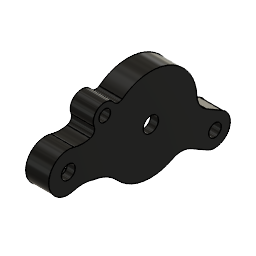
Dribbler Gear Cover v1 (Autodesk Fusion 360 design; units mm, degrees)
part number: 2026-04-20-20-56-39-992
Autodesk Fusion 360 part; units mm, degrees
sketch "Sketch1" plane through (0, 0, 0) normal (1, 0, 0) x (0, 0, -1)
  circle A0 centre (0, 0) radius 12
  circle A1 centre (0, 0) radius 2
  line L0 (0, 0) -> (-13.9, 0)
  circle A2 centre (-13.9, 0) radius 5.1
  line L1 (0, 0) -> (-21.5, 0)
  circle A3 centre (-21.5, 0) radius 5.1
  circle A4 centre (-21.5, 0) radius 1.8
  circle A5 centre (-13.9, 0) radius 1.75
  dimension "d1" = 24
  dimension "d3" = 4
  dimension "d4" = 13.9
  dimension "d5" = 10.2
  dimension "d6" = 21.5
  dimension "d7" = 10.2
  dimension "d8" = 3.6
  dimension "d9" = 3.5
  constraint coincident A0.centre A1.centre
  constraint horizontal L0
  constraint coincident L0.end A2.centre
  constraint parallel L0 L1
  constraint coincident L1.end A3.centre
  constraint concentric A3 A4
  constraint concentric A2 A5
  measures "d1" diameter of A0
  measures "d3" diameter of A1
  measures "d4" distance of A0.centre L0.end
  measures "d5" diameter of A2
  measures "d6" distance of A0.centre L1.end
  measures "d7" diameter of A3
  measures "d8" diameter of A4
  measures "d9" diameter of A5
extrude "Extrude1" add sketch "Sketch1" against normal blind 2 contours A0 A2 | A0 L0 A2 L1 | A0 L0 A2 L1 A3 A5 | A0 L0 A2 L1 A3 A5 | A0 L0 A2 L1 | A2 L1 A3 | A2 A3 | A2 L1 A3
extrude "Extrude2" add sketch "Sketch1" against normal blind 6 contours L0 L1 A5 | L0 L1 A5
fillet "Fillet1" radius 10 2 edges at (-1, 4.3231, 11.1942) (-1, -4.3231, 11.1942)
fillet "Fillet2" radius 8 2 edges at (-1, -3.4015, 17.7) (-1, 3.4015, 17.7)
sketch "Sketch2" plane through (-2, 0, 0) normal (-1, 0, 0) x (0, 0, 1)
  circle A0 centre (21.5, 0) radius 1.8
  circle A1 centre (13.9, 0) radius 1.75
  circle A2 centre (0, 0) radius 2
  arc A3 (15.3794, 4.8807) -> (14.6627, 5.0426) centre (13.9, 0) ccw
  arc A4 (8.8136, 8.1437) -> (14.6627, 5.0426) centre (16.1583, 14.9302) ccw
  arc A5 (8.8136, 8.1437) -> (8.8136, -8.1437) centre (0, 0) ccw
  arc A6 (14.6627, -5.0426) -> (8.8136, -8.1437) centre (16.1583, -14.9302) ccw
  arc A7 (14.6627, -5.0426) -> (15.3794, -4.8807) centre (13.9, 0) ccw
  arc A8 (20.0206, -4.8807) -> (15.3794, -4.8807) centre (17.7, -12.5367) ccw
  arc A9 (20.0206, -4.8807) -> (20.0206, 4.8807) centre (21.5, 0) ccw
  arc A10 (15.3794, 4.8807) -> (20.0206, 4.8807) centre (17.7, 12.5367) ccw
  circle A11 centre (0, 0) radius 11
  circle A12 centre (0, 0) radius 12
  circle A13 centre (13.9, 0) radius 4.6
  circle A14 centre (21.5, 0) radius 4.6
  circle A15 centre (13.9, 0) radius 5.1
  circle A16 centre (21.5, 0) radius 5.1
  dimension "d18" = 22
  dimension "d19" = 9.2
  dimension "d20" = 9.2
  dimension "d21" = 10.2
  dimension "d22" = 10.2
  constraint concentric A2 A11
  constraint concentric A11 A12
  constraint concentric A1 A13
  constraint concentric A0 A14
  constraint concentric A13 A15
  constraint concentric A14 A16
  measures "d18" diameter of A11
  measures "d19" diameter of A13
  measures "d20" diameter of A14
  measures "d21" diameter of A15
  measures "d22" diameter of A16
extrude "Extrude3" add sketch "Sketch2" along normal blind 4 contours A3 A12 A13 A15 A16 | A10 A15 A16 | A4 A12 A15 | A9 A14 A15 A16 | A5 A11 A12 A15 | A6 A12 A15 | A8 A15 A16 | A7 A12 A13 A15 A16
fillet "Fillet3" radius 4 1 edges at (-4, 3.6779, 10.3669)
fillet "Fillet4" radius 6 1 edges at (-4, 3.8409, 11.3687)
fillet "Fillet5" radius 4 1 edges at (-4, -3.6779, 10.3669)
fillet "Fillet6" radius 6 1 edges at (-4, -3.8409, 11.3687)
fillet "Fillet7" radius 15 4 edges at (-4, -3.0072, 17.3809) (-4, -3.0072, 18.0191) (-4, 3.0072, 17.3809) (-4, 3.0072, 18.0191)
sketch "Sketch3" plane through (0, 0, 0) normal (1, 0, 0) x (0, 0, -1)
  circle A0 centre (0, 0) radius 2
  circle A1 centre (-21.5, 0) radius 1.8
  arc A2 (-14.6627, 5.0426) -> (-15.3794, 4.8807) centre (-13.9, 0) ccw
  arc A3 (-20.0206, 4.8807) -> (-15.3794, 4.8807) centre (-17.7, 12.5367) ccw
  arc A4 (-20.0206, 4.8807) -> (-20.0206, -4.8807) centre (-21.5, 0) ccw
  arc A5 (-15.3794, -4.8807) -> (-20.0206, -4.8807) centre (-17.7, -12.5367) ccw
  arc A6 (-15.3794, -4.8807) -> (-14.6627, -5.0426) centre (-13.9, 0) ccw
  arc A7 (-8.8136, -8.1437) -> (-14.6627, -5.0426) centre (-16.1583, -14.9302) ccw
  arc A8 (-8.8136, -8.1437) -> (-8.8136, 8.1437) centre (0, 0) ccw
  arc A9 (-14.6627, 5.0426) -> (-8.8136, 8.1437) centre (-16.1583, 14.9302) ccw
  line L0 (0, 0) -> (-12, 0)
  line L1 (-12, 0) -> (-12, 8)
  circle A10 centre (-12, 8) radius 1.5
  circle A11 centre (-12, 8) radius 3
  dimension "d42" = 12
  dimension "d43" = 8
  dimension "d44" = 3
  dimension "d45" = 6
  constraint coincident A0.centre A8.centre
  constraint horizontal L0
  constraint perpendicular L0 L1
  constraint coincident L1.end A10.centre
  constraint concentric A10 A11
  measures "d42" distance of A0.centre L0.end
  measures "d43" distance of L0.end L1.end
  measures "d44" diameter of A10
  measures "d45" diameter of A11
extrude "Extrude4" add sketch "Sketch3" against normal blind 6 contours A9 A11
fillet "Fillet9" radius 1.5 2 edges at (-3, 5.3283, 13.3646) (-3, 7.9469, 9.0005)
fillet "Fillet10" radius 0.25 1 edges at (-6, 0.6328, 15.5316)
sketch "Sketch4" plane through (0, 0, 0) normal (1, 0, 0) x (0, 0, -1)
  circle A0 centre (-12, 8) radius 1.5
  circle A1 centre (0, 0) radius 2
  circle A2 centre (-21.5, 0) radius 1.8
  arc A3 (-15.7754, 4.7717) -> (-14.7575, 6.8184) centre (-16.1363, 6.2276) ccw
  arc A4 (-20.0206, 4.8807) -> (-15.7754, 4.7717) centre (-17.7, 12.5367) ccw
  arc A5 (-20.0206, 4.8807) -> (-20.0206, -4.8807) centre (-21.5, 0) ccw
  arc A6 (-15.3794, -4.8807) -> (-20.0206, -4.8807) centre (-17.7, -12.5367) ccw
  arc A7 (-15.3794, -4.8807) -> (-14.6627, -5.0426) centre (-13.9, 0) ccw
  arc A8 (-8.8136, -8.1437) -> (-14.6627, -5.0426) centre (-16.1583, -14.9302) ccw
  arc A9 (-8.8136, -8.1437) -> (-7.4124, 9.437) centre (0, 0) ccw
  arc A10 (-9.5593, 9.7444) -> (-7.4124, 9.437) centre (-8.3389, 10.6166) ccw
  arc A11 (-9.5593, 9.7444) -> (-14.7575, 6.8184) centre (-12, 8) ccw
  line L0 (0, 0) -> (16.7143, -9.65)
  line L1 (0, 0) -> (19.3, 0) construction
  circle A12 centre (16.7143, -9.65) radius 1.65
  circle A13 centre (16.7143, -9.65) radius 4
  line L2 (16.7143, -9.65) -> (18.7143, -6.1859)
  line L3 (18.7143, -6.1859) -> (11.798, -2.1928)
  line L4 (14.7262, -13.1209) -> (7.7759, -9.1398)
  dimension "d50" = 19.3
  dimension "d51" = 30
  dimension "d52" = 3.3
  dimension "d53" = 8
  constraint horizontal L1
  constraint coincident A1.centre A9.centre
  constraint coincident L0.end A12.centre
  constraint concentric A12 A13
  constraint coincident A13 L2.end
  constraint perpendicular L0 L2
  constraint coincident A9 L3.end
  constraint tangent A13 L3
  constraint coincident A13 L4.start
  constraint coincident A9 L4.end
  constraint tangent A13 L4
  measures "d50" distance of A1.centre L0.end
  measures "d51" angle of L0 L1
  measures "d52" diameter of A12
  measures "d53" diameter of A13
extrude "Extrude5" add sketch "Sketch4" against normal blind 6 contours A9 L0 A13 L3 | A9 L0 A13 L4 | L0 A12 A13 L2 | L0 A12 A13 L2
fillet "Fillet11" radius 5 2 edges at (-3, -2.1928, -11.798) (-3, -9.1398, -7.7759)
